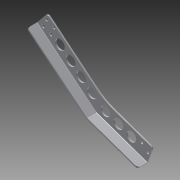
# Autodesk Inventor part: V5 Shooter Frame Channel P5
Saved by Autodesk Inventor 2014 SP1 (Build 180222100, 222)
## iProperties
Created: 2012-02-04
Part Number: V5 Shooter Frame Channel P5
Material: Aluminum-6061
Document SubType Name: Sheet Metal
Designer: Moses
Density: 2.71 g/cm^3
Sheet Metal Rule: Default
Mass: 130.216 g
Surface Area: 346.121 cm^2
Volume: 48.05 cm^3
Flat Pattern Width: 9.92395 cm
Flat Pattern Length: 30.0968 cm
Flat Pattern Area: 298.679 cm^2
Sheet Metal Width: 3.907 in
Sheet Metal Length: 11.849 in
Sheet Metal Area: 46.295 in^2
Appearance: Aluminum - Flat
Author: Moses
Autodesk Inventor part; units mm, degrees
ref_plane "YZ Plane" through (0, 0, 0) normal (1, 0, 0) x (0, 1, 0)
ref_plane "XZ Plane" through (0, 0, 0) normal (0, 1, 0) x (-1, 0, 0)
ref_plane "XY Plane" through (0, 0, 0) normal (0, 0, 1) x (1, 0, 0)
sketch "Sketch1" plane through (0, 0, 0) normal (0, 0, 1) x (1, 0, 0)
  arc A0 (11.5834, 105.2756) -> (11.5834, 96.2954) centre (16.0736, 100.7855) ccw construction
  line L0 (25.0538, 82.825) -> (11.5834, 96.2954) construction
  arc A1 (25.0538, 82.825) -> (34.0341, 82.825) centre (29.5439, 87.3151) ccw construction
  line L1 (55.0036, 103.7945) -> (34.0341, 82.825) construction
  line L2 (55.0036, 103.7945) -> (32.5529, 126.2451) construction
  line L3 (11.5834, 105.2756) -> (32.5529, 126.2451) construction
  circle A2 centre (20.5637, 105.2756) radius 3.3782 projected
  circle A3 centre (34.0341, 91.8052) radius 3.3782 projected
  arc A4 (-256.923, 48.7053) -> (-263.273, 55.0553) centre (-263.273, 48.7053) ccw construction
  line L4 (-282.323, 55.0553) -> (-263.273, 55.0553) construction
  arc A5 (-282.323, 55.0553) -> (-288.673, 48.7053) centre (-282.323, 48.7053) ccw construction
  line L5 (-288.673, 19.05) -> (-288.673, 48.7053) construction
  line L6 (-288.673, 19.05) -> (-256.923, 19.05) construction
  line L7 (-256.923, 48.7053) -> (-256.923, 19.05) construction
  circle A6 centre (-263.273, 42.3553) radius 3.3782 projected
  circle A7 centre (-282.323, 42.3553) radius 3.3782 projected
  arc A8 (15.875, 48.7053) -> (9.525, 55.0553) centre (9.525, 48.7053) ccw construction
  line L8 (-9.525, 55.0553) -> (9.525, 55.0553) construction
  arc A9 (-9.525, 55.0553) -> (-15.875, 48.7053) centre (-9.525, 48.7053) ccw construction
  line L9 (-15.875, 19.05) -> (-15.875, 48.7053) construction
  line L10 (-15.875, 19.05) -> (15.875, 19.05) construction
  line L11 (15.875, 48.7053) -> (15.875, 19.05) construction
  circle A10 centre (9.525, 42.3553) radius 3.3782 construction
  circle A11 centre (-9.525, 42.3553) radius 3.3782 construction
  arc A12 (-214.7543, 223.0847) -> (-213.0598, 218.9265) centre (-211.828, 221.8528) ccw construction
  line L12 (-189.6494, 209.072) -> (-213.0598, 218.9265) construction
  arc A13 (-189.6494, 209.072) -> (-185.4912, 210.7665) centre (-188.4175, 211.9983) ccw construction
  line L13 (-175.6367, 234.1769) -> (-185.4912, 210.7665) construction
  arc A14 (-175.6367, 234.1769) -> (-177.3312, 238.335) centre (-178.563, 235.4087) ccw construction
  line L14 (-200.7416, 248.1896) -> (-177.3312, 238.335) construction
  arc A15 (-200.7416, 248.1896) -> (-204.8997, 246.4951) centre (-201.9734, 245.2633) ccw construction
  line L15 (-214.7543, 223.0847) -> (-204.8997, 246.4951) construction
  circle A16 centre (-190.112, 216.1564) radius 3.3782 projected
  circle A17 centre (-207.6699, 223.5473) radius 3.3782 projected
  circle A18 centre (-182.7211, 233.7142) radius 3.3782 projected
  circle A19 centre (-200.2789, 241.1051) radius 3.3782 projected
  line L16 (45.9008, 106.4821) -> (-66.4223, 145.8093)
  line L17 (-80.1053, 132.1262) -> (64.3889, 276.6204) projected
  line L18 (-83.7757, 114.8814) -> (-220.3276, 226.6337)
  line L19 (-66.4223, 145.8093) -> (-198.2085, 253.6614)
  line L20 (-83.7757, 114.8814) -> (34.3596, 73.5192)
  line L21 (34.3596, 73.5192) -> (45.9008, 106.4821)
  line L22 (-220.3276, 226.6337) -> (-198.2085, 253.6614)
  line L23 (-182.7211, 233.7142) -> (-197.7114, 215.3974) construction
  line L24 (-197.7114, 215.3974) -> (-207.6699, 223.5473) construction
  line L25 (-220.3276, 226.6337) -> (-236.4143, 206.9772)
  line L26 (-236.4143, 206.9772) -> (-99.8624, 95.2248)
  line L27 (-83.7757, 114.8814) -> (-99.8624, 95.2248)
  line L28 (34.3596, 73.5192) -> (25.966, 49.5461)
  line L29 (25.966, 49.5461) -> (-92.1693, 90.9083)
  line L30 (-83.7757, 114.8814) -> (-92.1693, 90.9083)
  line L31 (-221.9363, 224.6681) -> (-85.3844, 112.9157) construction
  line L32 (-84.6151, 112.4841) -> (33.5203, 71.1219) construction
  line L33 (-212.9123, 215.6419) -> (-203.0841, 207.5986)
  line L34 (-212.9123, 215.6419) -> (-211.3037, 217.6075)
  line L35 (-211.3037, 217.6075) -> (-201.4754, 209.5642)
  line L36 (-201.4754, 209.5642) -> (-203.0841, 207.5986)
  line L37 (-191.4989, 198.1174) -> (-181.6706, 190.0741)
  line L38 (-191.4989, 198.1174) -> (-189.8903, 200.0831)
  line L39 (-189.8903, 200.0831) -> (-180.062, 192.0397)
  line L40 (-180.062, 192.0397) -> (-181.6706, 190.0741)
  line L41 (-170.0855, 180.593) -> (-160.2572, 172.5496)
  line L42 (-170.0855, 180.593) -> (-168.4768, 182.5586)
  line L43 (-168.4768, 182.5586) -> (-158.6486, 174.5153)
  line L44 (-158.6486, 174.5153) -> (-160.2572, 172.5496)
  line L45 (-148.6721, 163.0685) -> (-138.8438, 155.0252)
  line L46 (-148.6721, 163.0685) -> (-147.0634, 165.0341)
  line L47 (-147.0634, 165.0341) -> (-137.2351, 156.9908)
  line L48 (-137.2351, 156.9908) -> (-138.8438, 155.0252)
  line L49 (-127.2587, 145.544) -> (-117.4304, 137.5007)
  line L50 (-127.2587, 145.544) -> (-125.65, 147.5097)
  line L51 (-125.65, 147.5097) -> (-115.8217, 139.4663)
  line L52 (-115.8217, 139.4663) -> (-117.4304, 137.5007)
  line L53 (-105.8452, 128.0195) -> (-96.017, 119.9762)
  line L54 (-105.8452, 128.0195) -> (-104.2366, 129.9852)
  line L55 (-104.2366, 129.9852) -> (-94.4083, 121.9419)
  line L56 (-94.4083, 121.9419) -> (-96.017, 119.9762)
  line L57 (-73.0482, 107.0886) -> (-61.0617, 102.8918)
  line L58 (-73.0482, 107.0886) -> (-72.2088, 109.4859)
  line L59 (-72.2088, 109.4859) -> (-60.2223, 105.2891)
  line L60 (-60.2223, 105.2891) -> (-61.0617, 102.8918)
  line L61 (-52.5043, 99.8957) -> (-40.5177, 95.6989)
  line L62 (-52.5043, 99.8957) -> (-51.6649, 102.293)
  line L63 (-51.6649, 102.293) -> (-39.6784, 98.0962)
  line L64 (-39.6784, 98.0962) -> (-40.5177, 95.6989)
  line L65 (-31.9603, 92.7027) -> (-19.9738, 88.5059)
  line L66 (-31.9603, 92.7027) -> (-31.121, 95.1)
  line L67 (-31.121, 95.1) -> (-19.1345, 90.9032)
  line L68 (-19.1345, 90.9032) -> (-19.9738, 88.5059)
  line L69 (-11.4164, 85.5097) -> (0.5701, 81.3129)
  line L70 (-11.4164, 85.5097) -> (-10.5771, 87.907)
  line L71 (-10.5771, 87.907) -> (1.4095, 83.7103)
  line L72 (1.4095, 83.7103) -> (0.5701, 81.3129)
  line L73 (9.1275, 78.3168) -> (21.114, 74.12)
  line L74 (9.1275, 78.3168) -> (9.9669, 80.7141)
  line L75 (9.9669, 80.7141) -> (21.9534, 76.5173)
  line L76 (21.9534, 76.5173) -> (21.114, 74.12)
  line L77 (40.1302, 90.0006) -> (-75.099, 130.3453) construction
  line L78 (-75.099, 130.3453) -> (-209.268, 240.1476) construction
  circle A20 centre (-94.7555, 146.432) radius 11.1125
  circle A21 centre (-119.3262, 166.5403) radius 11.1125
  circle A22 centre (-143.8969, 186.6486) radius 11.1125
  circle A23 centre (-168.4675, 206.757) radius 11.1125
  circle A24 centre (-63.1124, 126.1485) radius 11.1125
  circle A25 centre (-33.1461, 115.6566) radius 11.1125
  circle A26 centre (-3.1798, 105.1646) radius 11.1125
  point P0 (0, 0)
  point P1 (-212.108, 216.6247)
  point P2 (-190.6946, 199.1003)
  point P3 (-169.2812, 181.5758)
  point P4 (-147.8677, 164.0513)
  point P5 (-126.4543, 146.5268)
  point P6 (-105.0409, 129.0024)
  point P7 (-72.6285, 108.2873)
  point P8 (-52.0846, 101.0943)
  point P9 (-31.5407, 93.9014)
  point P10 (-10.9967, 86.7084)
  point P11 (9.5472, 79.5154)
  dimension "d59" = 5.6281
  dimension "d60" = 6.35
  dimension "d67" = 160
  dimension "d70" = 6.35
  dimension "d72" = 34.925
  dimension "d73" = 34.925
  dimension "d74" = 5.6281
  dimension "d75" = 23.6688
  dimension "d76" = 25.4
  dimension "d77" = 25.4
  dimension "d78" = 2.54
  dimension "d80" = 2.54
  dimension "d93" = 12.7
  dimension "d94" = 2.54
  dimension "d95" = 12.7
  dimension "d96" = 176.4512
  dimension "d97" = 125.167
  dimension "d100" = 27.6702
  dimension "d105" = 12.7
  dimension "d106" = 2.54
  dimension "d107" = 12.7
  dimension "d110" = 21.7668
  dimension "d116" = 22.225
  dimension "d117" = 25.4
  dimension "d120" = 31.75
  dimension "d125" = 22.225
  dimension "d126" = 12.7
  dimension "d129" = 31.75
  constraints: 124 end point, 13 perpendicular, 11 point on line, 9 parallel, 7 centre point, 4 midpoint, 1 coincident, 1 collinear, 95 other
  measures "d59" distance from line of L19 A18.centre
  measures "d60" distance from line of L22 A19.centre
  measures "d67" angle of L20 L18
  measures "d70" distance from line of L21 A3.centre
  measures "d72" distance between parallel lines of L19 L18
  measures "d73" distance between parallel lines of L20 L16
  measures "d74" distance from line of L18 L24.end
  measures "d75" distance of L23.start L23.end
  measures "d76" distance of L18.end L25.end
  measures "d77" distance of L20.end L28.end
  measures "d78" distance between parallel lines of L18 L31
  measures "d80" distance between parallel lines of L20 L32
  measures "d93" distance of L33.start L33.end
  measures "d94" distance of L33.start L34.end
  measures "d95" distance between parallel lines of L25 L34
  measures "d96" distance of L31.start L31.end
  measures "d97" distance of L32.start L32.end
  measures "d100" distance of L33.start L38.start
  measures "d105" distance of L57.start L57.end
  measures "d106" distance of L57.start L58.end
  measures "d107" distance between parallel lines of L30 L58
  measures "d110" distance of L57.start L62.start
  measures "d116" diameter of A20
  measures "d117" distance of L77.end A20.centre
  measures "d120" distance of A20.centre A21.centre
  measures "d125" diameter of A24
  measures "d126" distance of L77.end A24.centre
  measures "d129" distance of A24.centre A25.centre
extrude "Plate1" add sketch "Sketch1" along normal blind 3.175 contours L21 L20 L18 L22 L19 L16 | L28 L29 L30 L20 | L27 L26 L25 L18 | L34 L35 L36 L33 | L38 L39 L40 L37 | L42 L43 L44 L41 | L46 L47 L48 L45 | L50 L51 L52 L49 | L54 L55 L56 L53 | L58 L59 L60 L57 | L62 L63 L64 L61 | L66 L67 L68 L65 | L70 L71 L72 L69 | L74 L75 L76 L73
fillet "Corner Round2" radius 127 1 edges at (-66.4223, 145.8093, 1.5875)
fold "Fold2" angle 90 bend radius 1.27 thickness 3.175 k factor 0.44 line from (-221.9363, 224.6681, 0) to (-85.3844, 112.9157, 0) line at bend centre moving side (-0.633333, -0.7738794, 0) folds toward (0, 0, 1)
fold "Fold3" angle 90 bend radius 1.27 thickness 3.175 k factor 0.44 line from (-84.6151, 112.4841, 0) to (33.5203, 71.1219, 0) line at bend centre moving side (-0.330456, -0.9438214, 0) folds toward (0, 0, 1)
fillet "Corner Round3" radius 6.35 4 edges at (-198.2085, 253.6614, 1.5875) (-222.4194, 224.0777, 25.2103) (33.2682, 70.4019, 25.2103) (45.9008, 106.4821, 1.5875)
equation "\"d59\" = -0.5 * d75 + 0.5 * d72"
equation "\"d70\" = d53"
equation "\"d73\" = d72"
equation "\"d80\" = d78"
equation "\"d100\" = -0.6 * d95 + 0.2 * d96"
equation "\"d107\" = d95"
equation "\"d110\" = -0.75 * d107 + 0.25 * d97"
equation "\"d81\" = BendReliefWidth"
equation "\"d82\" = BendReliefDepth"
equation "\"d83\" = MinimumRemnant"
equation "\"d84\" = BendRadius"
equation "\"d87\" = BendReliefWidth"
equation "\"d88\" = BendReliefDepth"
equation "\"d89\" = MinimumRemnant"
equation "\"d90\" = BendRadius"
equation "\"BendRadius\" = Thickness"
equation "\"BendReliefWidth\" = Thickness"
equation "\"BendReliefDepth\" = 0.5 * Thickness"
equation "\"CornerReliefSize\" = 4 * Thickness"
equation "\"MinimumRemnant\" = 2 * Thickness"
equation "\"TransitionRadius\" = BendRadius"
equation "\"JacobiRadiusSize\" = BendRadius"
equation "\"GapSize\" = Thickness"
equation "\"d5\" = BendRadius"
equation "\"d53\" = 6.35"
equation "\"Thickness\" = 3.175"
body "Solid1"
